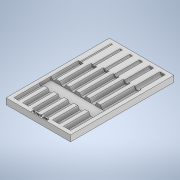
# Autodesk Inventor part: punchTray
Saved by Autodesk Inventor 2020.2 (Build 242310000, 310)
## iProperties
Created: 2019-12-07
Part Number: punchTray
Material: Generic
Document SubType Name: Modeling
Designer: robst
Density: 1 g/cm^3
Appearance: Default
Author: robst
Autodesk Inventor part; units mm, degrees
(part 1 of 2)
ref_plane "YZ Plane" through (0, 0, 0) normal (1, 0, 0) x (0, 1, 0)
ref_plane "XZ Plane" through (0, 0, 0) normal (0, 1, 0) x (-1, 0, 0)
ref_plane "XY Plane" through (0, 0, 0) normal (0, 0, 1) x (1, 0, 0)
sketch "Sketch3" plane through (0, 0, 0) normal (0, 0, 1) x (1, 0, 0)
  line L0 (-52.4636, -4.8895) -> (52.4636, -4.8895)
  line L1 (52.4636, -4.8895) -> (52.4636, 4.8895)
  line L2 (52.4636, 4.8895) -> (-52.4636, 4.8895)
  line L3 (-52.4636, 4.8895) -> (-52.4636, -4.8895)
  line L4 (-52.4636, -4.8895) -> (52.4636, 4.8895) construction
  line L5 (52.4636, -4.8895) -> (-52.4636, 4.8895) construction
  line L6 (46.1136, 4.8895) -> (43.2173, -0.127)
  line L7 (43.2173, -0.127) -> (37.4248, -0.127)
  line L8 (37.4248, -0.127) -> (34.5285, 4.8895)
  line L9 (34.5285, 4.8895) -> (37.4248, 9.906)
  line L10 (37.4248, 9.906) -> (43.2173, 9.906)
  line L11 (43.2173, 9.906) -> (46.1136, 4.8895)
  line L12 (28.1785, 4.8895) -> (25.2822, -0.127)
  line L13 (25.2822, -0.127) -> (19.4897, -0.127)
  line L14 (19.4897, -0.127) -> (16.5934, 4.8895)
  line L15 (16.5934, 4.8895) -> (19.4897, 9.906)
  line L16 (19.4897, 9.906) -> (25.2822, 9.906)
  line L17 (25.2822, 9.906) -> (28.1785, 4.8895)
  line L18 (0, 0) -> (0, 4.8895) construction
  line L19 (10.2434, 4.8895) -> (7.787, 0.635)
  line L20 (7.787, 0.635) -> (2.8744, 0.635)
  line L21 (2.8744, 0.635) -> (0.418, 4.8895)
  line L22 (0.418, 4.8895) -> (2.8744, 9.144)
  line L23 (2.8744, 9.144) -> (7.787, 9.144)
  line L24 (7.787, 9.144) -> (10.2434, 4.8895)
  line L25 (-5.932, 4.8895) -> (-8.3883, 0.635)
  line L26 (-8.3883, 0.635) -> (-13.301, 0.635)
  line L27 (-13.301, 0.635) -> (-15.7573, 4.8895)
  line L28 (-15.7573, 4.8895) -> (-13.301, 9.144)
  line L29 (-13.301, 9.144) -> (-8.3883, 9.144)
  line L30 (-8.3883, 9.144) -> (-5.932, 4.8895)
  line L31 (-22.1073, 4.8895) -> (-24.5416, 0.6731)
  line L32 (-24.5416, 0.6731) -> (-29.4103, 0.6731)
  line L33 (-29.4103, 0.6731) -> (-31.8447, 4.8895)
  line L34 (-31.8447, 4.8895) -> (-29.4103, 9.1059)
  line L35 (-29.4103, 9.1059) -> (-24.5416, 9.1059)
  line L36 (-24.5416, 9.1059) -> (-22.1073, 4.8895)
  line L37 (-38.1947, 4.8895) -> (-40.1744, 1.4605)
  line L38 (-40.1744, 1.4605) -> (-44.1339, 1.4605)
  line L39 (-44.1339, 1.4605) -> (-46.1136, 4.8895)
  line L40 (-46.1136, 4.8895) -> (-44.1339, 8.3185)
  line L41 (-44.1339, 8.3185) -> (-40.1744, 8.3185)
  line L42 (-40.1744, 8.3185) -> (-38.1947, 4.8895)
  point P0 (40.321, 4.8895)
  point P1 (22.3859, 4.8895)
  point P2 (34.5285, 4.8895)
  point P3 (16.5934, 4.8895)
  point P4 (5.3307, 4.8895)
  point P5 (-10.8446, 4.8895)
  point P6 (-26.976, 4.8895)
  point P7 (-42.1541, 4.8895)
  point P8 (0.418, 4.8895)
  point P9 (-15.7573, 4.8895)
  point P10 (-31.8447, 4.8895)
  point P11 (-46.1136, 4.8895)
  dimension "d7" = 10.033
  dimension "d8" = 10.033
  dimension "d13" = 6.35
  dimension "d14" = 6.35
  dimension "d15" = 8.509
  dimension "d16" = 6.35
  dimension "d17" = 8.509
  dimension "d18" = 6.35
  dimension "d19" = 8.4328
  dimension "d20" = 6.35
  dimension "d21" = 6.35
  dimension "d22" = 6.858
  dimension "d23" = 6.35
  dimension "d24" = 4.7625
  constraints: 84 end point, 2 horizontal, 2 midpoint, 1 parallel, 1 perpendicular, 94 other
  measures "d7" distance between parallel lines of L7 L10
  measures "d8" distance between parallel lines of L13 L16
  measures "d13" distance of L6.start L1.end
  measures "d14" distance of L8.end L12.start
  measures "d15" distance between parallel lines of L20 L23
  measures "d16" distance of L14.end L19.start
  measures "d17" distance between parallel lines of L26 L29
  measures "d18" distance of L21.end L25.start
  measures "d19" distance between parallel lines of L32 L35
  measures "d20" distance of L27.end L31.start
  measures "d21" distance of L33.end L37.start
  measures "d22" distance between parallel lines of L38 L41
  measures "d23" distance from line of L39.end L3
  measures "d24" distance between parallel lines of L0 L7
extrude "Extrusion3" add sketch "Sketch3" against normal blind 155.575 contours L3 L2 L39 L38 L37 L33 L32 L31 L27 L26 L25 L21 L20 L19 L14 L13 L12 L8 L7 L6 L1 L0
sketch "Sketch4" plane through (0, 0, 0) normal (0, 0, 1) x (1, 0, 0)
  line L0 (52.4636, -4.8895) -> (-52.4636, -4.8895) projected
  line L1 (52.4636, 4.8895) -> (52.4636, -4.8895) projected
  line L2 (-52.4636, -4.8895) -> (52.4636, -4.8895)
  line L3 (52.4636, -4.8895) -> (52.4636, 4.8895)
  line L4 (52.4636, 4.8895) -> (-52.4636, 4.8895)
  line L5 (-52.4636, 4.8895) -> (-52.4636, -4.8895)
  point P0 (0, 0)
  constraints: 8 end point, 2 parallel, 1 horizontal, 1 perpendicular
extrude "Extrusion4" add sketch "Sketch4" along normal blind 6.35
sketch "Sketch6" plane through (0, 0, -155.575) normal (0, 0, -1) x (-1, 0, 0)
  line L0 (-37.4248, -0.127) -> (-43.2173, -0.127) construction
  line L1 (-40.321, -0.127) -> (-40.321, 4.8895) construction
  line L2 (-52.4636, 4.8895) -> (52.4636, 4.8895) construction
  arc A0 (-44.5438, 4.8895) -> (-36.0983, 4.8895) centre (-40.321, 4.8895) ccw
  line L3 (-34.5285, 4.8895) -> (-37.4248, -0.127)
  line L4 (-37.4248, -0.127) -> (-43.2173, -0.127)
  line L5 (-43.2173, -0.127) -> (-46.1136, 4.8895)
  line L6 (-46.1136, 4.8895) -> (-44.5438, 4.8895)
  line L7 (-34.5285, 4.8895) -> (-36.0983, 4.8895)
  point P0 (0, 0)
  dimension "d31" = 8.4455
  constraints: 12 end point, 3 point on line, 2 coincident, 2 point on circle, 1 centre point, 1 midpoint, 1 vertical, 6 other
  measures "d31" diameter of A0
extrude "5_16_punch" add sketch "Sketch6" against normal blind 40.64
sketch "Sketch7" plane through (0, 0, -155.575) normal (0, 0, -1) x (-1, 0, 0)
  line L0 (-28.1785, 4.8895) -> (-16.5934, 4.8895) projected
  line L1 (-16.5934, 4.8895) -> (-19.4897, -0.127)
  line L2 (-19.4897, -0.127) -> (-25.2822, -0.127)
  line L3 (-25.2822, -0.127) -> (-28.1785, 4.8895)
  arc A0 (-25.8149, 4.8895) -> (-18.9569, 4.8895) centre (-22.3859, 4.8895) ccw
  line L4 (-28.1785, 4.8895) -> (-25.8149, 4.8895)
  line L5 (-10.2434, 4.8895) -> (-16.5934, 4.8895) projected
  line L6 (-16.5934, 4.8895) -> (-18.9569, 4.8895)
  point P0 (0, 0)
  point P1 (-28.1785, 4.8895)
  dimension "d34" = 6.858
  constraints: 10 end point, 2 point on circle, 2 point on line, 1 centre point, 1 coincident, 1 midpoint, 6 other
  measures "d34" diameter of A0
extrude "1_4_punch" add sketch "Sketch7" against normal blind 40.64 contours L0 A0 L1 L2 L3
sketch "Sketch8" plane through (0, 0, -155.575) normal (0, 0, -1) x (-1, 0, 0)
  line L0 (-10.2434, 4.8895) -> (-0.418, 4.8895) projected
  line L1 (-0.418, 4.8895) -> (-2.8744, 0.635)
  line L2 (-2.8744, 0.635) -> (-7.787, 0.635)
  line L3 (-7.787, 0.635) -> (-10.2434, 4.8895)
  arc A0 (-7.966, 4.8895) -> (-2.6955, 4.8895) centre (-5.3307, 4.8895) ccw
  line L4 (-10.2434, 4.8895) -> (-7.787, 0.635) projected
  line L5 (-10.2434, 4.8895) -> (-7.966, 4.8895)
  line L6 (-0.418, 4.8895) -> (-2.6955, 4.8895)
  point P0 (0, 0)
  dimension "d37" = 5.2705
  constraints: 10 end point, 2 point on circle, 2 point on line, 1 centre point, 1 coincident, 1 midpoint, 6 other
  measures "d37" diameter of A0
extrude "3_16_punch" add sketch "Sketch8" against normal blind 40.64 contours L0 A0 L1 L2 L3
sketch "Sketch9" plane through (0, 0, -155.575) normal (0, 0, -1) x (-1, 0, 0)
  line L0 (13.301, 0.635) -> (8.3883, 0.635) construction
  line L1 (10.8446, 0.635) -> (10.8446, 4.8895) construction
  line L2 (-52.4636, 4.8895) -> (52.4636, 4.8895) construction
  line L3 (15.7573, 4.8895) -> (13.301, 0.635) projected
  line L4 (15.7573, 4.8895) -> (13.301, 0.635)
  line L5 (13.301, 0.635) -> (8.3883, 0.635)
  line L6 (8.3883, 0.635) -> (5.932, 4.8895)
  arc A0 (8.6063, 4.8895) -> (13.083, 4.8895) centre (10.8446, 4.8895) ccw
  line L7 (8.3883, 0.635) -> (5.932, 4.8895) projected
  line L8 (5.932, 4.8895) -> (8.6063, 4.8895)
  line L9 (22.1073, 4.8895) -> (15.7573, 4.8895) projected
  line L10 (15.7573, 4.8895) -> (13.083, 4.8895)
  point P0 (0, 0)
  point P1 (13.301, 0.635)
  dimension "d40" = 4.4768
  constraints: 12 end point, 3 point on line, 2 coincident, 2 point on circle, 1 centre point, 1 midpoint, 1 vertical, 6 other
  measures "d40" diameter of A0
extrude "5_32_punch" add sketch "Sketch9" against normal blind 40.64
sketch "Sketch11" plane through (0, 0, -155.575) normal (0, 0, -1) x (-1, 0, 0)
  line L0 (22.1073, 4.8895) -> (31.8447, 4.8895) projected
  line L1 (29.4103, 0.6731) -> (31.8447, 4.8895) projected
  line L2 (31.8447, 4.8895) -> (29.4103, 0.6731)
  line L3 (29.4103, 0.6731) -> (24.5416, 0.6731)
  line L4 (24.5416, 0.6731) -> (22.1073, 4.8895)
  arc A0 (25.1345, 4.8895) -> (28.8175, 4.8895) centre (26.976, 4.8895) ccw
  line L5 (22.1073, 4.8895) -> (24.5416, 0.6731) projected
  line L6 (22.1073, 4.8895) -> (25.1345, 4.8895)
  line L7 (31.8447, 4.8895) -> (28.8175, 4.8895)
  point P0 (0, 0)
  point P1 (29.4103, 0.6731)
  point P2 (22.1073, 4.8895)
  dimension "d44" = 3.683
  constraints: 10 end point, 2 point on circle, 2 point on line, 1 centre point, 1 coincident, 1 midpoint, 6 other
  measures "d44" diameter of A0
extrude "1_8_punch" add sketch "Sketch11" against normal blind 44.45 contours L0 A0 L1 L3 L4
sketch "Sketch12" plane through (0, 0, -155.575) normal (0, 0, -1) x (-1, 0, 0)
  line L0 (40.1744, 1.4605) -> (44.1339, 1.4605) construction
  line L1 (42.1541, 1.4605) -> (42.1541, 4.8895) construction
  line L2 (-52.4636, 4.8895) -> (52.4636, 4.8895) construction
  line L3 (44.1339, 1.4605) -> (46.1136, 4.8895) projected
  line L4 (46.1136, 4.8895) -> (44.1339, 1.4605)
  line L5 (44.1339, 1.4605) -> (40.1744, 1.4605)
  line L6 (40.1744, 1.4605) -> (38.1947, 4.8895)
  arc A0 (41.1064, 4.8895) -> (43.2019, 4.8895) centre (42.1541, 4.8895) ccw
  line L7 (38.1947, 4.8895) -> (28.8175, 4.8895) projected
  line L8 (38.1947, 4.8895) -> (41.1064, 4.8895)
  line L9 (46.1136, 4.8895) -> (43.2019, 4.8895)
  point P0 (0, 0)
  point P1 (44.1339, 1.4605)
  dimension "d47" = 2.0955
  constraints: 12 end point, 3 point on line, 2 coincident, 2 point on circle, 1 centre point, 1 midpoint, 1 vertical, 6 other
  measures "d47" diameter of A0
extrude "1_16_punch" add sketch "Sketch12" against normal blind 50.8
sketch "Sketch5" plane through (0, 0, -155.575) normal (0, 0, -1) x (-1, 0, 0)
  line L0 (-52.4636, 4.8895) -> (-52.4636, -4.8895) projected
  line L1 (52.4636, 4.8895) -> (46.1136, 4.8895) projected
  line L2 (-52.4636, -4.8895) -> (52.4636, -4.8895)
  line L3 (52.4636, -4.8895) -> (52.4636, 4.8895)
  line L4 (52.4636, 4.8895) -> (-52.4636, 4.8895)
  line L5 (-52.4636, 4.8895) -> (-52.4636, -4.8895)
  point P0 (0, 0)
  constraints: 8 end point, 2 parallel, 1 horizontal, 1 perpendicular
extrude "Extrusion5" add sketch "Sketch5" along normal blind 6.35
sketch "Sketch13" plane through (-52.4636, 4.8895, 6.35) normal (0, 1, 0) x (1, 0, 0)
  line L0 (6.35, 6.35) -> (6.35, 111.125) projected
  line L1 (98.5772, 6.35) -> (98.5772, 121.285) projected
  line L2 (6.35, 47.625) -> (98.5772, 47.625)
  line L3 (98.5772, 47.625) -> (98.5772, 66.675)
  line L4 (98.5772, 66.675) -> (6.35, 66.675)
  line L5 (6.35, 66.675) -> (6.35, 47.625)
  line L6 (6.35, 57.15) -> (98.5772, 57.15) construction
  line L7 (14.2689, 6.35) -> (6.35, 6.35) construction
  point P0 (52.4636, 6.35)
  point P1 (6.35, 66.675)
  dimension "d50" = 19.05
  dimension "d51" = 50.8
  constraints: 10 end point, 2 midpoint, 2 parallel, 2 point on line, 1 horizontal, 1 perpendicular
  measures "d50" distance between parallel lines of L4 L2
  measures "d51" distance between parallel lines of L6 L7
extrude "Extrusion12" cut sketch "Sketch13" against normal blind 5.08
sketch "Sketch14" plane through (-52.4636, 4.8895, 6.35) normal (0, 1, 0) x (1, 0, 0)
  line L0 (0, 168.275) -> (0, 0) construction
  line L1 (0, 3.175) -> (104.9272, 3.175) construction
  line L2 (0, 0) -> (104.9272, 0) construction
  spline S0 degree 2 poles (42.5851, 3.879) (42.5851, 3.6134) (42.4153, 3.1318) (42.2578, 2.9712) knots 0 0 0 1 2 2 2
  spline S1 degree 2 poles (42.2578, 2.9712) (42.1621, 2.8693) (41.9274, 2.7026) (41.7885, 2.6439) knots 0 0 0 1 2 2 2
  spline S2 degree 2 poles (41.7885, 2.6439) (41.6465, 2.5853) (41.3161, 2.5174) (41.1123, 2.5174) knots 0 0 0 1 2 2 2
  line L3 (41.1123, 2.5174) -> (40.6122, 2.5174)
  line L4 (40.6122, 2.5174) -> (40.6122, 1.27)
  line L5 (40.6122, 1.27) -> (39.655, 1.27)
  line L6 (39.655, 1.27) -> (39.655, 5.08)
  line L7 (39.655, 5.08) -> (41.1339, 5.08)
  spline S3 degree 2 poles (41.1339, 5.08) (41.4612, 5.08) (41.9398, 4.9596) (42.1343, 4.8299) knots 0 0 0 1 2 2 2
  spline S4 degree 2 poles (42.1343, 4.8299) (42.3504, 4.6848) (42.5851, 4.2093) (42.5851, 3.879) knots 0 0 0 1 2 2 2
  spline S5 degree 2 poles (41.6033, 3.8543) (41.6033, 4.0179) (41.4489, 4.2495) (41.3439, 4.2927) knots 0 0 0 1 2 2 2
  spline S6 degree 2 poles (41.3439, 4.2927) (41.208, 4.3513) (40.961, 4.3699) (40.748, 4.3699) knots 0 0 0 1 2 2 2
  line L8 (40.748, 4.3699) -> (40.6122, 4.3699)
  line L9 (40.6122, 4.3699) -> (40.6122, 3.2275)
  line L10 (40.6122, 3.2275) -> (40.6801, 3.2275)
  spline S7 degree 2 poles (40.6801, 3.2275) (40.8128, 3.2275) (41.0537, 3.2337) (41.1432, 3.2491) knots 0 0 0 1 2 2 2
  spline S8 degree 2 poles (41.1432, 3.2491) (41.2204, 3.2615) (41.3902, 3.3356) (41.4365, 3.3819) knots 0 0 0 1 2 2 2
  spline S9 degree 2 poles (41.4365, 3.3819) (41.5353, 3.4745) (41.6033, 3.6814) (41.6033, 3.8543) knots 0 0 0 1 2 2 2
  line L11 (45.7127, 1.27) -> (44.8174, 1.27)
  line L12 (44.8174, 1.27) -> (44.8174, 1.588)
  spline S10 degree 2 poles (44.8174, 1.588) (44.5858, 1.3935) (44.1968, 1.1897) (43.9282, 1.1897) knots 0 0 0 1 2 2 2
  spline S11 degree 2 poles (43.9282, 1.1897) (43.5021, 1.1897) (43.0235, 1.73) (43.0235, 2.2734) knots 0 0 0 1 2 2 2
  line L13 (43.0235, 2.2734) -> (43.0235, 4.1445)
  line L14 (43.0235, 4.1445) -> (43.9251, 4.1445)
  line L15 (43.9251, 4.1445) -> (43.9251, 2.718)
  spline S12 degree 2 poles (43.9251, 2.718) (43.9251, 2.4957) (43.9467, 2.2117) (43.9899, 2.116) knots 0 0 0 1 2 2 2
  spline S13 degree 2 poles (43.9899, 2.116) (44.0331, 2.0264) (44.2029, 1.9338) (44.3573, 1.9338) knots 0 0 0 1 2 2 2
  spline S14 degree 2 poles (44.3573, 1.9338) (44.4499, 1.9338) (44.7093, 2.0264) (44.8174, 2.1067) knots 0 0 0 1 2 2 2
  line L16 (44.8174, 2.1067) -> (44.8174, 4.1445)
  line L17 (44.8174, 4.1445) -> (45.7127, 4.1445)
  line L18 (45.7127, 4.1445) -> (45.7127, 1.27)
  line L19 (49.0874, 1.27) -> (48.1858, 1.27)
  line L20 (48.1858, 1.27) -> (48.1858, 2.6933)
  spline S15 degree 2 poles (48.1858, 2.6933) (48.1858, 2.8693) (48.1581, 3.2151) (48.121, 3.2954) knots 0 0 0 1 2 2 2
  spline S16 degree 2 poles (48.121, 3.2954) (48.0747, 3.3942) (47.9018, 3.4776) (47.7536, 3.4776) knots 0 0 0 1 2 2 2
  spline S17 degree 2 poles (47.7536, 3.4776) (47.6455, 3.4776) (47.4201, 3.3942) (47.2936, 3.3047) knots 0 0 0 1 2 2 2
  line L21 (47.2936, 3.3047) -> (47.2936, 1.27)
  line L22 (47.2936, 1.27) -> (46.3982, 1.27)
  line L23 (46.3982, 1.27) -> (46.3982, 4.1445)
  line L24 (46.3982, 4.1445) -> (47.2936, 4.1445)
  line L25 (47.2936, 4.1445) -> (47.2936, 3.8265)
  spline S18 degree 2 poles (47.2936, 3.8265) (47.5128, 4.0117) (47.9296, 4.2217) (48.1828, 4.2217) knots 0 0 0 1 2 2 2
  spline S19 degree 2 poles (48.1828, 4.2217) (48.6212, 4.2217) (49.0874, 3.6659) (49.0874, 3.141) knots 0 0 0 1 2 2 2
  line L26 (49.0874, 3.141) -> (49.0874, 1.27)
  spline S20 degree 2 poles (51.1591, 1.1928) (50.8041, 1.1928) (50.2143, 1.3719) (49.9951, 1.5571) knots 0 0 0 1 2 2 2
  spline S21 degree 2 poles (49.9951, 1.5571) (49.7821, 1.7455) (49.5413, 2.3105) (49.5413, 2.6933) knots 0 0 0 1 2 2 2
  spline S22 degree 2 poles (49.5413, 2.6933) (49.5413, 3.1071) (49.8006, 3.6844) (50.026, 3.8697) knots 0 0 0 1 2 2 2
  spline S23 degree 2 poles (50.026, 3.8697) (50.239, 4.0488) (50.8195, 4.2217) (51.1344, 4.2217) knots 0 0 0 1 2 2 2
  spline S24 degree 2 poles (51.1344, 4.2217) (51.3722, 4.2217) (51.8476, 4.1105) (52.0885, 3.9901) knots 0 0 0 1 2 2 2
  line L27 (52.0885, 3.9901) -> (52.0885, 3.2244)
  line L28 (52.0885, 3.2244) -> (51.9742, 3.2244)
  spline S25 degree 2 poles (51.9742, 3.2244) (51.9187, 3.2769) (51.7643, 3.4004) (51.6717, 3.4498) knots 0 0 0 1 2 2 2
  spline S26 degree 2 poles (51.6717, 3.4498) (51.5729, 3.5054) (51.3289, 3.5795) (51.1777, 3.5795) knots 0 0 0 1 2 2 2
  spline S27 degree 2 poles (51.1777, 3.5795) (50.8349, 3.5795) (50.4583, 3.1009) (50.4583, 2.6933) knots 0 0 0 1 2 2 2
  spline S28 degree 2 poles (50.4583, 2.6933) (50.4583, 2.2611) (50.8596, 1.835) (51.1931, 1.835) knots 0 0 0 1 2 2 2
  spline S29 degree 2 poles (51.1931, 1.835) (51.3629, 1.835) (51.6161, 1.9122) (51.7087, 1.9678) knots 0 0 0 1 2 2 2
  spline S30 degree 2 poles (51.7087, 1.9678) (51.7982, 2.0203) (51.9279, 2.1376) (51.9742, 2.1839) knots 0 0 0 1 2 2 2
  line L29 (51.9742, 2.1839) -> (52.0885, 2.1839)
  line L30 (52.0885, 2.1839) -> (52.0885, 1.4151)
  spline S31 degree 2 poles (52.0885, 1.4151) (52.0113, 1.3812) (51.8106, 1.2947) (51.7056, 1.2669) knots 0 0 0 1 2 2 2
  spline S32 degree 2 poles (51.7056, 1.2669) (51.5759, 1.2299) (51.3475, 1.1928) (51.1591, 1.1928) knots 0 0 0 1 2 2 2
  line L31 (55.2038, 1.27) -> (54.3022, 1.27)
  line L32 (54.3022, 1.27) -> (54.3022, 2.6933)
  spline S33 degree 2 poles (54.3022, 2.6933) (54.3022, 2.8693) (54.2744, 3.2151) (54.2374, 3.2954) knots 0 0 0 1 2 2 2
  spline S34 degree 2 poles (54.2374, 3.2954) (54.1911, 3.3942) (54.0182, 3.4776) (53.87, 3.4776) knots 0 0 0 1 2 2 2
  spline S35 degree 2 poles (53.87, 3.4776) (53.7619, 3.4776) (53.5365, 3.3942) (53.4099, 3.3047) knots 0 0 0 1 2 2 2
  line L33 (53.4099, 3.3047) -> (53.4099, 1.27)
  line L34 (53.4099, 1.27) -> (52.5145, 1.27)
  line L35 (52.5145, 1.27) -> (52.5145, 5.2498)
  line L36 (52.5145, 5.2498) -> (53.4099, 5.2498)
  line L37 (53.4099, 5.2498) -> (53.4099, 3.8265)
  spline S36 degree 2 poles (53.4099, 3.8265) (53.6291, 4.0117) (54.046, 4.2217) (54.2991, 4.2217) knots 0 0 0 1 2 2 2
  spline S37 degree 2 poles (54.2991, 4.2217) (54.7376, 4.2217) (55.2038, 3.6659) (55.2038, 3.141) knots 0 0 0 1 2 2 2
  line L38 (55.2038, 3.141) -> (55.2038, 1.27)
  spline S38 degree 2 poles (58.6309, 1.2021) (58.1925, 1.2021) (57.5318, 1.3719) (57.2477, 1.4954) knots 0 0 0 1 2 2 2
  line L39 (57.2477, 1.4954) -> (57.2477, 2.4031)
  line L40 (57.2477, 2.4031) -> (57.3342, 2.4031)
  spline S39 degree 2 poles (57.3342, 2.4031) (57.6213, 2.1592) (58.3098, 1.8968) (58.634, 1.8968) knots 0 0 0 1 2 2 2
  spline S40 degree 2 poles (58.634, 1.8968) (58.7174, 1.8968) (58.986, 1.9338) (59.0663, 1.9709) knots 0 0 0 1 2 2 2
  spline S41 degree 2 poles (59.0663, 1.9709) (59.1651, 2.0141) (59.304, 2.1716) (59.304, 2.2981) knots 0 0 0 1 2 2 2
  spline S42 degree 2 poles (59.304, 2.2981) (59.304, 2.4433) (59.0786, 2.6223) (58.9242, 2.6625) knots 0 0 0 1 2 2 2
  spline S43 degree 2 poles (58.9242, 2.6625) (58.7297, 2.715) (58.2882, 2.8045) (58.0937, 2.8724) knots 0 0 0 1 2 2 2
  spline S44 degree 2 poles (58.0937, 2.8724) (57.6522, 3.0268) (57.2693, 3.5548) (57.2693, 3.95) knots 0 0 0 1 2 2 2
  spline S45 degree 2 poles (57.2693, 3.95) (57.2693, 4.4841) (58.174, 5.1479) (58.8532, 5.1479) knots 0 0 0 1 2 2 2
  spline S46 degree 2 poles (58.8532, 5.1479) (59.1929, 5.1479) (59.8659, 5.009) (60.1315, 4.8917) knots 0 0 0 1 2 2 2
  line L41 (60.1315, 4.8917) -> (60.1315, 4.021)
  line L42 (60.1315, 4.021) -> (60.0481, 4.021)
  spline S47 degree 2 poles (60.0481, 4.021) (59.8351, 4.2031) (59.2237, 4.4532) (58.9026, 4.4532) knots 0 0 0 1 2 2 2
  spline S48 degree 2 poles (58.9026, 4.4532) (58.776, 4.4532) (58.5784, 4.4162) (58.4673, 4.3668) knots 0 0 0 1 2 2 2
  spline S49 degree 2 poles (58.4673, 4.3668) (58.3778, 4.3266) (58.2481, 4.1661) (58.2481, 4.0673) knots 0 0 0 1 2 2 2
  spline S50 degree 2 poles (58.2481, 4.0673) (58.2481, 3.9191) (58.4549, 3.7493) (58.7513, 3.6814) knots 0 0 0 1 2 2 2
  spline S51 degree 2 poles (58.7513, 3.6814) (58.9428, 3.6381) (59.2978, 3.5548) (59.5016, 3.4838) knots 0 0 0 1 2 2 2
  spline S52 degree 2 poles (59.5016, 3.4838) (59.8968, 3.3386) (60.2828, 2.857) (60.2828, 2.4618) knots 0 0 0 1 2 2 2
  spline S53 degree 2 poles (60.2828, 2.4618) (60.2828, 1.8937) (59.3905, 1.2021) (58.6309, 1.2021) knots 0 0 0 1 2 2 2
  spline S54 degree 2 poles (62.1939, 1.1928) (61.3788, 1.1928) (60.5112, 1.9709) (60.5112, 2.6903) knots 0 0 0 1 2 2 2
  spline S55 degree 2 poles (60.5112, 2.6903) (60.5112, 3.3942) (61.3202, 4.234) (62.0488, 4.234) knots 0 0 0 1 2 2 2
  spline S56 degree 2 poles (62.0488, 4.234) (62.7065, 4.234) (63.3734, 3.5208) (63.3734, 2.8601) knots 0 0 0 1 2 2 2
  line L43 (63.3734, 2.8601) -> (63.3734, 2.5359)
  line L44 (63.3734, 2.5359) -> (61.4066, 2.5359)
  spline S57 degree 2 poles (61.4066, 2.5359) (61.419, 2.3352) (61.5641, 2.0697) (61.6814, 1.9894) knots 0 0 0 1 2 2 2
  spline S58 degree 2 poles (61.6814, 1.9894) (61.7956, 1.9091) (62.1044, 1.8412) (62.2866, 1.8412) knots 0 0 0 1 2 2 2
  spline S59 degree 2 poles (62.2866, 1.8412) (62.4409, 1.8412) (62.7435, 1.9091) (62.8701, 1.9678) knots 0 0 0 1 2 2 2
  spline S60 degree 2 poles (62.8701, 1.9678) (62.9812, 2.0141) (63.1665, 2.1283) (63.2252, 2.1716) knots 0 0 0 1 2 2 2
  line L45 (63.2252, 2.1716) -> (63.3209, 2.1716)
  line L46 (63.3209, 2.1716) -> (63.3209, 1.4306)
  spline S61 degree 2 poles (63.3209, 1.4306) (63.2097, 1.3873) (63.0306, 1.3132) (62.8701, 1.2762) knots 0 0 0 1 2 2 2
  spline S62 degree 2 poles (62.8701, 1.2762) (62.725, 1.236) (62.4162, 1.1928) (62.1939, 1.1928) knots 0 0 0 1 2 2 2
  spline S63 degree 2 poles (62.4903, 3.0762) (62.4842, 3.3603) (62.2341, 3.6597) (61.9778, 3.6597) knots 0 0 0 1 2 2 2
  spline S64 degree 2 poles (61.9778, 3.6597) (61.7154, 3.6597) (61.419, 3.3448) (61.4035, 3.0762) knots 0 0 0 1 2 2 2
  line L47 (61.4035, 3.0762) -> (62.4903, 3.0762)
  spline S65 degree 2 poles (64.9326, 1.2144) (64.3861, 1.2144) (63.8859, 1.6652) (63.8859, 2.1777) knots 0 0 0 1 2 2 2
  line L48 (63.8859, 2.1777) -> (63.8859, 3.5208)
  line L49 (63.8859, 3.5208) -> (63.5432, 3.5208)
  line L50 (63.5432, 3.5208) -> (63.5432, 4.1445)
  line L51 (63.5432, 4.1445) -> (63.8859, 4.1445)
  line L52 (63.8859, 4.1445) -> (63.8859, 4.9658)
  line L53 (63.8859, 4.9658) -> (64.7813, 4.9658)
  line L54 (64.7813, 4.9658) -> (64.7813, 4.1445)
  line L55 (64.7813, 4.1445) -> (65.6458, 4.1445)
  line L56 (65.6458, 4.1445) -> (65.6458, 3.5208)
  line L57 (65.6458, 3.5208) -> (64.7813, 3.5208)
  line L58 (64.7813, 3.5208) -> (64.7813, 2.4988)
  spline S66 degree 2 poles (64.7813, 2.4988) (64.7813, 2.3475) (64.7874, 2.1222) (64.8245, 2.0326) knots 0 0 0 1 2 2 2
  spline S67 degree 2 poles (64.8245, 2.0326) (64.8615, 1.9431) (65.0437, 1.8381) (65.2166, 1.8381) knots 0 0 0 1 2 2 2
  spline S68 degree 2 poles (65.2166, 1.8381) (65.2907, 1.8381) (65.5223, 1.8999) (65.5686, 1.9246) knots 0 0 0 1 2 2 2
  line L59 (65.5686, 1.9246) -> (65.6458, 1.9246)
  line L60 (65.6458, 1.9246) -> (65.6458, 1.2947)
  spline S69 degree 2 poles (65.6458, 1.2947) (65.5007, 1.2576) (65.1734, 1.2144) (64.9326, 1.2144) knots 0 0 0 1 2 2 2
  point P0 (52.4636, 6.35)
  dimension "d54" = 3.175
  constraints: 2 end point, 1 horizontal, 1 parallel, 1 point on line
  measures "d54" distance between parallel lines of L1 L2
extrude "Extrusion13" cut sketch "Sketch14" against normal blind 3.175
sketch "Sketch15" plane through (-52.4636, -4.8895, 6.35) normal (0, -1, 0) x (1, 0, 0)
  line L0 (104.9272, -168.275) -> (104.9272, 0) construction
  line L1 (104.9272, -84.1375) -> (0, -84.1375) construction
  line L2 (0, -168.275) -> (0, 0) construction
  spline S0 degree 2 poles (77.1638, -95.5613) (77.1638, -94.493) (78.0962, -92.8134) (78.8063, -92.3627) knots 0 0 0 1 2 2 2
  spline S1 degree 2 poles (78.8063, -92.3627) (79.3991, -91.9798) (80.7947, -91.7575) (81.5789, -91.7575) knots 0 0 0 1 2 2 2
  line L3 (81.5789, -91.7575) -> (83.9625, -91.7575)
  line L4 (83.9625, -91.7575) -> (83.9625, -99.3775)
  line L5 (83.9625, -99.3775) -> (81.6036, -99.3775)
  spline S2 degree 2 poles (81.6036, -99.3775) (80.8009, -99.3775) (79.3991, -99.1737) (78.7816, -98.7785) knots 0 0 0 1 2 2 2
  spline S3 degree 2 poles (78.7816, -98.7785) (78.0344, -98.2969) (77.1638, -96.6667) (77.1638, -95.5613) knots 0 0 0 1 2 2 2
  spline S4 degree 2 poles (79.1274, -95.5737) (79.1274, -96.327) (79.6461, -97.4015) (80.1772, -97.7041) knots 0 0 0 1 2 2 2
  spline S5 degree 2 poles (80.1772, -97.7041) (80.5662, -97.914) (81.4184, -97.9572) (82.0112, -97.9572) knots 0 0 0 1 2 2 2
  line L6 (82.0112, -97.9572) -> (82.0482, -97.9572)
  line L7 (82.0482, -97.9572) -> (82.0482, -93.1839)
  line L8 (82.0482, -93.1839) -> (82.0112, -93.1839)
  spline S6 degree 2 poles (82.0112, -93.1839) (81.369, -93.1839) (80.4859, -93.2272) (80.0846, -93.4803) knots 0 0 0 1 2 2 2
  spline S7 degree 2 poles (80.0846, -93.4803) (79.6153, -93.7767) (79.1274, -94.8203) (79.1274, -95.5737) knots 0 0 0 1 2 2 2
  spline S8 degree 2 poles (73.187, -91.6031) (74.8173, -91.6031) (76.5524, -93.1592) (76.5524, -94.598) knots 0 0 0 1 2 2 2
  spline S9 degree 2 poles (76.5524, -94.598) (76.5524, -96.0059) (74.9346, -97.6855) (73.4773, -97.6855) knots 0 0 0 1 2 2 2
  spline S10 degree 2 poles (73.4773, -97.6855) (72.162, -97.6855) (70.8282, -96.2591) (70.8282, -94.9376) knots 0 0 0 1 2 2 2
  line L9 (70.8282, -94.9376) -> (70.8282, -94.2893)
  line L10 (70.8282, -94.2893) -> (74.7617, -94.2893)
  spline S11 degree 2 poles (74.7617, -94.2893) (74.737, -93.8879) (74.4467, -93.3568) (74.2121, -93.1963) knots 0 0 0 1 2 2 2
  spline S12 degree 2 poles (74.2121, -93.1963) (73.9836, -93.0357) (73.3661, -92.8999) (73.0018, -92.8999) knots 0 0 0 1 2 2 2
  spline S13 degree 2 poles (73.0018, -92.8999) (72.693, -92.8999) (72.0879, -93.0357) (71.8347, -93.1531) knots 0 0 0 1 2 2 2
  spline S14 degree 2 poles (71.8347, -93.1531) (71.6124, -93.2457) (71.2419, -93.4742) (71.1246, -93.5606) knots 0 0 0 1 2 2 2
  line L11 (71.1246, -93.5606) -> (70.9332, -93.5606)
  line L12 (70.9332, -93.5606) -> (70.9332, -92.0786)
  spline S15 degree 2 poles (70.9332, -92.0786) (71.1555, -91.9922) (71.5136, -91.844) (71.8347, -91.7699) knots 0 0 0 1 2 2 2
  spline S16 degree 2 poles (71.8347, -91.7699) (72.1249, -91.6896) (72.7424, -91.6031) (73.187, -91.6031) knots 0 0 0 1 2 2 2
  spline S17 degree 2 poles (72.5942, -95.3699) (72.6066, -95.938) (73.1068, -96.537) (73.6193, -96.537) knots 0 0 0 1 2 2 2
  spline S18 degree 2 poles (73.6193, -96.537) (74.1442, -96.537) (74.737, -95.9071) (74.7679, -95.3699) knots 0 0 0 1 2 2 2
  line L13 (74.7679, -95.3699) -> (72.5942, -95.3699)
  spline S19 degree 2 poles (68.1606, -91.6031) (68.7904, -91.6031) (69.9204, -91.881) (70.2909, -92.0663) knots 0 0 0 1 2 2 2
  line L14 (70.2909, -92.0663) -> (70.2909, -93.5791)
  line L15 (70.2909, -93.5791) -> (70.1427, -93.5791)
  spline S20 degree 2 poles (70.1427, -93.5791) (70.0131, -93.4803) (69.6858, -93.2457) (69.3956, -93.116) knots 0 0 0 1 2 2 2
  spline S21 degree 2 poles (69.3956, -93.116) (69.1424, -92.9987) (68.5187, -92.832) (68.1482, -92.832) knots 0 0 0 1 2 2 2
  spline S22 degree 2 poles (68.1482, -92.832) (67.7715, -92.832) (67.1911, -93.0666) (67.1911, -93.3198) knots 0 0 0 1 2 2 2
  spline S23 degree 2 poles (67.1911, -93.3198) (67.1911, -93.5174) (67.4566, -93.7273) (67.8395, -93.8138) knots 0 0 0 1 2 2 2
  spline S24 degree 2 poles (67.8395, -93.8138) (68.0432, -93.8694) (68.6669, -93.9867) (68.9077, -94.0608) knots 0 0 0 1 2 2 2
  spline S25 degree 2 poles (68.9077, -94.0608) (69.587, -94.2707) (70.2662, -95.092) (70.2662, -95.7651) knots 0 0 0 1 2 2 2
  spline S26 degree 2 poles (70.2662, -95.7651) (70.2662, -96.148) (69.9143, -96.8272) (69.5685, -97.0927) knots 0 0 0 1 2 2 2
  spline S27 degree 2 poles (69.5685, -97.0927) (69.2288, -97.3521) (68.2223, -97.6608) (67.5863, -97.6608) knots 0 0 0 1 2 2 2
  spline S28 degree 2 poles (67.5863, -97.6608) (66.9811, -97.6608) (65.9684, -97.42) (65.6226, -97.2533) knots 0 0 0 1 2 2 2
  line L16 (65.6226, -97.2533) -> (65.6226, -95.796)
  line L17 (65.6226, -95.796) -> (65.7646, -95.796)
  spline S29 degree 2 poles (65.7646, -95.796) (65.8573, -95.8701) (66.2586, -96.1109) (66.4439, -96.1974) knots 0 0 0 1 2 2 2
  spline S30 degree 2 poles (66.4439, -96.1974) (66.6724, -96.2962) (67.2281, -96.432) (67.5184, -96.432) knots 0 0 0 1 2 2 2
  spline S31 degree 2 poles (67.5184, -96.432) (67.9074, -96.432) (68.4446, -96.1665) (68.4446, -95.9504) knots 0 0 0 1 2 2 2
  spline S32 degree 2 poles (68.4446, -95.9504) (68.4446, -95.7528) (68.1791, -95.5304) (67.7345, -95.4193) knots 0 0 0 1 2 2 2
  spline S33 degree 2 poles (67.7345, -95.4193) (67.506, -95.3637) (66.907, -95.2587) (66.6291, -95.1661) knots 0 0 0 1 2 2 2
  spline S34 degree 2 poles (66.6291, -95.1661) (66.0116, -94.9685) (65.3694, -94.1966) (65.3694, -93.5544) knots 0 0 0 1 2 2 2
  spline S35 degree 2 poles (65.3694, -93.5544) (65.3694, -93.1531) (65.7461, -92.4182) (66.0981, -92.1712) knots 0 0 0 1 2 2 2
  spline S36 degree 2 poles (66.0981, -92.1712) (66.4624, -91.8995) (67.4628, -91.6031) (68.1606, -91.6031) knots 0 0 0 1 2 2 2
  line L18 (62.7265, -91.7575) -> (64.5173, -91.7575)
  line L19 (64.5173, -91.7575) -> (64.5173, -97.5065)
  line L20 (64.5173, -97.5065) -> (62.7265, -97.5065)
  line L21 (62.7265, -97.5065) -> (62.7265, -91.7575)
  line L22 (62.6709, -98.3277) -> (64.5667, -98.3277)
  line L23 (64.5667, -98.3277) -> (64.5667, -99.7233)
  line L24 (64.5667, -99.7233) -> (62.6709, -99.7233)
  line L25 (62.6709, -99.7233) -> (62.6709, -98.3277)
  spline S37 degree 2 poles (56.1316, -92.4182) (56.1316, -91.6216) (56.5947, -90.504) (56.9899, -90.1952) knots 0 0 0 1 2 2 2
  spline S38 degree 2 poles (56.9899, -90.1952) (57.3913, -89.8803) (58.5028, -89.5962) (59.182, -89.5962) knots 0 0 0 1 2 2 2
  spline S39 degree 2 poles (59.182, -89.5962) (59.7563, -89.5962) (60.7876, -89.7444) (61.1642, -89.8432) knots 0 0 0 1 2 2 2
  line L26 (61.1642, -89.8432) -> (61.1642, -91.282)
  line L27 (61.1642, -91.282) -> (60.9543, -91.282)
  spline S40 degree 2 poles (60.9543, -91.282) (60.8246, -91.2326) (60.4603, -91.1091) (60.275, -91.0597) knots 0 0 0 1 2 2 2
  spline S41 degree 2 poles (60.275, -91.0597) (60.0527, -91.0041) (59.6328, -90.93) (59.4167, -90.93) knots 0 0 0 1 2 2 2
  spline S42 degree 2 poles (59.4167, -90.93) (58.9597, -90.93) (58.3546, -91.1153) (58.2002, -91.2882) knots 0 0 0 1 2 2 2
  spline S43 degree 2 poles (58.2002, -91.2882) (58.0458, -91.4673) (57.9223, -91.9489) (57.9223, -92.3194) knots 0 0 0 1 2 2 2
  line L28 (57.9223, -92.3194) -> (57.9223, -92.4244)
  spline S44 degree 2 poles (57.9223, -92.4244) (58.2249, -92.1589) (59.0153, -91.8378) (59.4352, -91.8378) knots 0 0 0 1 2 2 2
  spline S45 degree 2 poles (59.4352, -91.8378) (60.5529, -91.8378) (61.7632, -93.2889) (61.7632, -94.7771) knots 0 0 0 1 2 2 2
  spline S46 degree 2 poles (61.7632, -94.7771) (61.7632, -95.4502) (61.3927, -96.5246) (61.0593, -96.9013) knots 0 0 0 1 2 2 2
  spline S47 degree 2 poles (61.0593, -96.9013) (60.7382, -97.2656) (59.8428, -97.6608) (59.355, -97.6608) knots 0 0 0 1 2 2 2
  spline S48 degree 2 poles (59.355, -97.6608) (58.9165, -97.6608) (58.2187, -97.4385) (57.9347, -97.2533) knots 0 0 0 1 2 2 2
  line L29 (57.9347, -97.2533) -> (57.8668, -97.5065)
  line L30 (57.8668, -97.5065) -> (56.1316, -97.5065)
  line L31 (56.1316, -97.5065) -> (56.1316, -92.4182)
  line L32 (57.9223, -93.5668) -> (57.9223, -96.1727)
  spline S49 degree 2 poles (57.9223, -96.1727) (58.052, -96.2344) (58.441, -96.3147) (58.6386, -96.3147) knots 0 0 0 1 2 2 2
  spline S50 degree 2 poles (58.6386, -96.3147) (59.2809, -96.3147) (59.9292, -95.481) (59.9292, -94.7339) knots 0 0 0 1 2 2 2
  spline S51 degree 2 poles (59.9292, -94.7339) (59.9292, -94.3634) (59.8304, -93.8447) (59.7008, -93.6471) knots 0 0 0 1 2 2 2
  spline S52 degree 2 poles (59.7008, -93.6471) (59.5711, -93.4495) (59.1573, -93.2519) (58.8362, -93.2519) knots 0 0 0 1 2 2 2
  spline S53 degree 2 poles (58.8362, -93.2519) (58.5954, -93.2519) (58.1323, -93.4186) (57.9223, -93.5668) knots 0 0 0 1 2 2 2
  line L33 (49.3823, -91.7575) -> (51.1854, -91.7575)
  line L34 (51.1854, -91.7575) -> (51.1854, -94.6042)
  spline S54 degree 2 poles (51.1854, -94.6042) (51.1854, -94.9562) (51.2409, -95.6478) (51.315, -95.8083) knots 0 0 0 1 2 2 2
  spline S55 degree 2 poles (51.315, -95.8083) (51.4077, -96.0059) (51.7535, -96.1727) (52.0499, -96.1727) knots 0 0 0 1 2 2 2
  spline S56 degree 2 poles (52.0499, -96.1727) (52.266, -96.1727) (52.7168, -96.0059) (52.97, -95.8269) knots 0 0 0 1 2 2 2
  line L35 (52.97, -95.8269) -> (52.97, -91.7575)
  line L36 (52.97, -91.7575) -> (54.7607, -91.7575)
  line L37 (54.7607, -91.7575) -> (54.7607, -97.5065)
  line L38 (54.7607, -97.5065) -> (52.97, -97.5065)
  line L39 (52.97, -97.5065) -> (52.97, -96.8704)
  spline S57 degree 2 poles (52.97, -96.8704) (52.5315, -97.2409) (51.6979, -97.6608) (51.1915, -97.6608) knots 0 0 0 1 2 2 2
  spline S58 degree 2 poles (51.1915, -97.6608) (50.3147, -97.6608) (49.3823, -96.5493) (49.3823, -95.4996) knots 0 0 0 1 2 2 2
  line L40 (49.3823, -95.4996) -> (49.3823, -91.7575)
  spline S59 degree 2 poles (45.1091, -91.6031) (46.7393, -91.6031) (48.4745, -93.1592) (48.4745, -94.598) knots 0 0 0 1 2 2 2
  spline S60 degree 2 poles (48.4745, -94.598) (48.4745, -96.0059) (46.8567, -97.6855) (45.3994, -97.6855) knots 0 0 0 1 2 2 2
  spline S61 degree 2 poles (45.3994, -97.6855) (44.0841, -97.6855) (42.7503, -96.2591) (42.7503, -94.9376) knots 0 0 0 1 2 2 2
  line L41 (42.7503, -94.9376) -> (42.7503, -94.2893)
  line L42 (42.7503, -94.2893) -> (46.6838, -94.2893)
  spline S62 degree 2 poles (46.6838, -94.2893) (46.6591, -93.8879) (46.3688, -93.3568) (46.1342, -93.1963) knots 0 0 0 1 2 2 2
  spline S63 degree 2 poles (46.1342, -93.1963) (45.9057, -93.0357) (45.2882, -92.8999) (44.9239, -92.8999) knots 0 0 0 1 2 2 2
  spline S64 degree 2 poles (44.9239, -92.8999) (44.6151, -92.8999) (44.01, -93.0357) (43.7568, -93.1531) knots 0 0 0 1 2 2 2
  spline S65 degree 2 poles (43.7568, -93.1531) (43.5345, -93.2457) (43.164, -93.4742) (43.0467, -93.5606) knots 0 0 0 1 2 2 2
  line L43 (43.0467, -93.5606) -> (42.8552, -93.5606)
  line L44 (42.8552, -93.5606) -> (42.8552, -92.0786)
  spline S66 degree 2 poles (42.8552, -92.0786) (43.0775, -91.9922) (43.4357, -91.844) (43.7568, -91.7699) knots 0 0 0 1 2 2 2
  spline S67 degree 2 poles (43.7568, -91.7699) (44.047, -91.6896) (44.6645, -91.6031) (45.1091, -91.6031) knots 0 0 0 1 2 2 2
  spline S68 degree 2 poles (44.5163, -95.3699) (44.5287, -95.938) (45.0289, -96.537) (45.5414, -96.537) knots 0 0 0 1 2 2 2
  spline S69 degree 2 poles (45.5414, -96.537) (46.0663, -96.537) (46.6591, -95.9071) (46.6899, -95.3699) knots 0 0 0 1 2 2 2
  line L45 (46.6899, -95.3699) -> (44.5163, -95.3699)
  line L46 (36.6061, -91.7575) -> (38.3969, -91.7575)
  line L47 (38.3969, -91.7575) -> (38.3969, -92.3565)
  spline S70 degree 2 poles (38.3969, -92.3565) (38.5698, -92.2145) (39.0144, -91.8872) (39.1873, -91.8007) knots 0 0 0 1 2 2 2
  spline S71 degree 2 poles (39.1873, -91.8007) (39.3972, -91.7019) (39.8171, -91.5969) (40.1073, -91.5969) knots 0 0 0 1 2 2 2
  spline S72 degree 2 poles (40.1073, -91.5969) (41.0892, -91.5969) (42.2377, -93.2272) (42.2377, -94.5857) knots 0 0 0 1 2 2 2
  spline S73 degree 2 poles (42.2377, -94.5857) (42.2377, -95.339) (41.8487, -96.4444) (41.5091, -96.8519) knots 0 0 0 1 2 2 2
  spline S74 degree 2 poles (41.5091, -96.8519) (41.1942, -97.2286) (40.305, -97.6608) (39.8109, -97.6608) knots 0 0 0 1 2 2 2
  spline S75 degree 2 poles (39.8109, -97.6608) (39.3602, -97.6608) (38.7797, -97.4694) (38.3969, -97.2718) knots 0 0 0 1 2 2 2
  line L48 (38.3969, -97.2718) -> (38.3969, -99.7171)
  line L49 (38.3969, -99.7171) -> (36.6061, -99.7171)
  line L50 (36.6061, -99.7171) -> (36.6061, -91.7575)
  line L51 (38.3969, -93.3383) -> (38.3969, -96.1603)
  spline S76 degree 2 poles (38.3969, -96.1603) (38.5265, -96.2282) (38.9588, -96.3147) (39.1132, -96.3147) knots 0 0 0 1 2 2 2
  spline S77 degree 2 poles (39.1132, -96.3147) (39.7554, -96.3147) (40.4038, -95.4131) (40.4038, -94.6042) knots 0 0 0 1 2 2 2
  spline S78 degree 2 poles (40.4038, -94.6042) (40.4038, -93.752) (39.885, -92.9925) (39.3108, -92.9925) knots 0 0 0 1 2 2 2
  spline S79 degree 2 poles (39.3108, -92.9925) (39.0761, -92.9925) (38.5945, -93.1778) (38.3969, -93.3383) knots 0 0 0 1 2 2 2
  spline S80 degree 2 poles (26.5346, -94.7092) (26.5346, -93.3383) (27.924, -91.6463) (28.9552, -91.6463) knots 0 0 0 1 2 2 2
  spline S81 degree 2 poles (28.9552, -91.6463) (29.3813, -91.6463) (30.0173, -91.8378) (30.3755, -92.0416) knots 0 0 0 1 2 2 2
  line L52 (30.3755, -92.0416) -> (30.4496, -91.7575)
  line L53 (30.4496, -91.7575) -> (32.1662, -91.7575)
  line L54 (32.1662, -91.7575) -> (32.1662, -99.7171)
  line L55 (32.1662, -99.7171) -> (30.3755, -99.7171)
  line L56 (30.3755, -99.7171) -> (30.3755, -96.9013)
  spline S82 degree 2 poles (30.3755, -96.9013) (29.9803, -97.2409) (29.1652, -97.6608) (28.6279, -97.6608) knots 0 0 0 1 2 2 2
  spline S83 degree 2 poles (28.6279, -97.6608) (27.6214, -97.6608) (26.5346, -96.0986) (26.5346, -94.7092) knots 0 0 0 1 2 2 2
  spline S84 degree 2 poles (28.3686, -94.6721) (28.3686, -95.5304) (28.8873, -96.2653) (29.4307, -96.2653) knots 0 0 0 1 2 2 2
  spline S85 degree 2 poles (29.4307, -96.2653) (29.6715, -96.2653) (30.147, -96.1109) (30.3755, -95.9565) knots 0 0 0 1 2 2 2
  line L57 (30.3755, -95.9565) -> (30.3755, -93.079)
  spline S86 degree 2 poles (30.3755, -93.079) (30.1964, -93.0049) (29.8321, -92.9555) (29.653, -92.9555) knots 0 0 0 1 2 2 2
  spline S87 degree 2 poles (29.653, -92.9555) (29.0046, -92.9555) (28.3686, -93.8138) (28.3686, -94.6721) knots 0 0 0 1 2 2 2
  line L58 (20.1867, -97.5065) -> (23.0828, -89.6518)
  line L59 (23.0828, -89.6518) -> (25.0094, -89.6518)
  line L60 (25.0094, -89.6518) -> (24.1387, -91.8995)
  line L61 (24.1387, -91.8995) -> (26.2444, -97.5065)
  line L62 (26.2444, -97.5065) -> (24.3672, -97.5065)
  line L63 (24.3672, -97.5065) -> (23.1569, -93.9002)
  line L64 (23.1569, -93.9002) -> (22.0268, -97.5065)
  line L65 (22.0268, -97.5065) -> (20.1867, -97.5065)
  line L66 (72.9277, -78.9951) -> (75.2557, -78.9951)
  line L67 (75.2557, -78.9951) -> (77.3737, -81.7924)
  line L68 (77.3737, -81.7924) -> (78.0653, -81.7924)
  line L69 (78.0653, -81.7924) -> (78.0653, -78.9951)
  line L70 (78.0653, -78.9951) -> (79.9672, -78.9951)
  line L71 (79.9672, -78.9951) -> (79.9672, -86.6151)
  line L72 (79.9672, -86.6151) -> (76.9044, -86.6151)
  spline S88 degree 2 poles (76.9044, -86.6151) (76.2684, -86.6151) (75.3298, -86.4545) (74.9284, -86.2075) knots 0 0 0 1 2 2 2
  spline S89 degree 2 poles (74.9284, -86.2075) (74.5209, -85.9482) (74.0392, -85.1392) (74.0392, -84.5217) knots 0 0 0 1 2 2 2
  spline S90 degree 2 poles (74.0392, -84.5217) (74.0392, -83.651) (74.8296, -82.5581) (75.4903, -82.237) knots 0 0 0 1 2 2 2
  line L73 (75.4903, -82.237) -> (72.9277, -78.9951)
  spline S91 degree 2 poles (76.0029, -84.2809) (76.0029, -84.5711) (76.2252, -84.9849) (76.4783, -85.096) knots 0 0 0 1 2 2 2
  spline S92 degree 2 poles (76.4783, -85.096) (76.6574, -85.1701) (77.0958, -85.2133) (77.4231, -85.2133) knots 0 0 0 1 2 2 2
  line L74 (77.4231, -85.2133) -> (78.0653, -85.2133)
  line L75 (78.0653, -85.2133) -> (78.0653, -83.1632)
  line L76 (78.0653, -83.1632) -> (77.5157, -83.1632)
  spline S93 degree 2 poles (77.5157, -83.1632) (77.1205, -83.1632) (76.5586, -83.262) (76.3672, -83.4164) knots 0 0 0 1 2 2 2
  spline S94 degree 2 poles (76.3672, -83.4164) (76.1819, -83.5646) (76.0029, -83.9598) (76.0029, -84.2809) knots 0 0 0 1 2 2 2
  spline S95 degree 2 poles (66.9503, -81.8665) (66.9503, -80.4462) (68.5002, -78.816) (69.9143, -78.816) knots 0 0 0 1 2 2 2
  spline S96 degree 2 poles (69.9143, -78.816) (71.3222, -78.816) (72.8845, -80.4462) (72.8845, -81.8665) knots 0 0 0 1 2 2 2
  spline S97 degree 2 poles (72.8845, -81.8665) (72.8845, -83.2991) (71.3222, -84.9231) (69.9143, -84.9231) knots 0 0 0 1 2 2 2
  spline S98 degree 2 poles (69.9143, -84.9231) (68.5064, -84.9231) (66.9503, -83.2929) (66.9503, -81.8665) knots 0 0 0 1 2 2 2
  spline S99 degree 2 poles (68.7842, -81.8541) (68.7842, -82.3666) (68.951, -83.0521) (69.0992, -83.2558) knots 0 0 0 1 2 2 2
  spline S100 degree 2 poles (69.0992, -83.2558) (69.2597, -83.472) (69.6611, -83.6387) (69.9143, -83.6387) knots 0 0 0 1 2 2 2
  spline S101 degree 2 poles (69.9143, -83.6387) (70.1613, -83.6387) (70.5503, -83.4905) (70.7109, -83.2805) knots 0 0 0 1 2 2 2
  spline S102 degree 2 poles (70.7109, -83.2805) (70.8652, -83.0829) (71.0505, -82.3852) (71.0505, -81.8541) knots 0 0 0 1 2 2 2
  spline S103 degree 2 poles (71.0505, -81.8541) (71.0505, -81.3292) (70.8776, -80.6809) (70.7356, -80.4833) knots 0 0 0 1 2 2 2
  spline S104 degree 2 poles (70.7356, -80.4833) (70.5935, -80.2856) (70.1613, -80.1004) (69.9019, -80.1004) knots 0 0 0 1 2 2 2
  spline S105 degree 2 poles (69.9019, -80.1004) (69.6858, -80.1004) (69.2412, -80.2856) (69.1053, -80.4709) knots 0 0 0 1 2 2 2
  spline S106 degree 2 poles (69.1053, -80.4709) (68.951, -80.687) (68.7842, -81.3107) (68.7842, -81.8541) knots 0 0 0 1 2 2 2
  spline S107 degree 2 poles (60.3677, -81.9467) (60.3677, -80.5759) (61.757, -78.8839) (62.7883, -78.8839) knots 0 0 0 1 2 2 2
  spline S108 degree 2 poles (62.7883, -78.8839) (63.2144, -78.8839) (63.8504, -79.0753) (64.2085, -79.2791) knots 0 0 0 1 2 2 2
  line L77 (64.2085, -79.2791) -> (64.2826, -78.9951)
  line L78 (64.2826, -78.9951) -> (65.9993, -78.9951)
  line L79 (65.9993, -78.9951) -> (65.9993, -86.9547)
  line L80 (65.9993, -86.9547) -> (64.2085, -86.9547)
  line L81 (64.2085, -86.9547) -> (64.2085, -84.1389)
  spline S109 degree 2 poles (64.2085, -84.1389) (63.8133, -84.4785) (62.9982, -84.8984) (62.461, -84.8984) knots 0 0 0 1 2 2 2
  spline S110 degree 2 poles (62.461, -84.8984) (61.4545, -84.8984) (60.3677, -83.3361) (60.3677, -81.9467) knots 0 0 0 1 2 2 2
  spline S111 degree 2 poles (62.2016, -81.9097) (62.2016, -82.768) (62.7203, -83.5028) (63.2638, -83.5028) knots 0 0 0 1 2 2 2
  spline S112 degree 2 poles (63.2638, -83.5028) (63.5046, -83.5028) (63.9801, -83.3485) (64.2085, -83.1941) knots 0 0 0 1 2 2 2
  line L82 (64.2085, -83.1941) -> (64.2085, -80.3165)
  spline S113 degree 2 poles (64.2085, -80.3165) (64.0295, -80.2424) (63.6651, -80.193) (63.4861, -80.193) knots 0 0 0 1 2 2 2
  spline S114 degree 2 poles (63.4861, -80.193) (62.8377, -80.193) (62.2016, -81.0514) (62.2016, -81.9097) knots 0 0 0 1 2 2 2
  spline S115 degree 2 poles (53.853, -78.8592) (54.7298, -78.8592) (56.0513, -79.1988) (56.6194, -79.4458) knots 0 0 0 1 2 2 2
  line L83 (56.6194, -79.4458) -> (56.6194, -81.2613)
  line L84 (56.6194, -81.2613) -> (56.4465, -81.2613)
  spline S116 degree 2 poles (56.4465, -81.2613) (55.8722, -80.7735) (54.4952, -80.2486) (53.8468, -80.2486) knots 0 0 0 1 2 2 2
  spline S117 degree 2 poles (53.8468, -80.2486) (53.6801, -80.2486) (53.1429, -80.3227) (52.9823, -80.3968) knots 0 0 0 1 2 2 2
  spline S118 degree 2 poles (52.9823, -80.3968) (52.7847, -80.4833) (52.5068, -80.7982) (52.5068, -81.0514) knots 0 0 0 1 2 2 2
  spline S119 degree 2 poles (52.5068, -81.0514) (52.5068, -81.3416) (52.9576, -81.6997) (53.2664, -81.78) knots 0 0 0 1 2 2 2
  spline S120 degree 2 poles (53.2664, -81.78) (53.6554, -81.885) (54.5384, -82.0641) (54.9274, -82.1999) knots 0 0 0 1 2 2 2
  spline S121 degree 2 poles (54.9274, -82.1999) (55.8105, -82.5087) (56.5762, -83.5646) (56.5762, -84.355) knots 0 0 0 1 2 2 2
  spline S122 degree 2 poles (56.5762, -84.355) (56.5762, -85.4233) (54.7669, -86.7509) (53.4084, -86.7509) knots 0 0 0 1 2 2 2
  spline S123 degree 2 poles (53.4084, -86.7509) (52.7291, -86.7509) (51.383, -86.473) (50.8519, -86.2384) knots 0 0 0 1 2 2 2
  line L85 (50.8519, -86.2384) -> (50.8519, -84.497)
  line L86 (50.8519, -84.497) -> (51.0186, -84.497)
  spline S124 degree 2 poles (51.0186, -84.497) (51.4447, -84.8614) (52.6674, -85.3615) (53.3096, -85.3615) knots 0 0 0 1 2 2 2
  spline S125 degree 2 poles (53.3096, -85.3615) (53.5628, -85.3615) (53.958, -85.2874) (54.1803, -85.1886) knots 0 0 0 1 2 2 2
  spline S126 degree 2 poles (54.1803, -85.1886) (54.3593, -85.1084) (54.6187, -84.7873) (54.6187, -84.5897) knots 0 0 0 1 2 2 2
  spline S127 degree 2 poles (54.6187, -84.5897) (54.6187, -84.2933) (54.205, -83.9536) (53.6122, -83.8178) knots 0 0 0 1 2 2 2
  spline S128 degree 2 poles (53.6122, -83.8178) (53.2293, -83.7313) (52.5192, -83.5646) (52.1116, -83.4226) knots 0 0 0 1 2 2 2
  spline S129 degree 2 poles (52.1116, -83.4226) (51.3212, -83.1323) (50.5493, -82.169) (50.5493, -81.3786) knots 0 0 0 1 2 2 2
  spline S130 degree 2 poles (50.5493, -81.3786) (50.5493, -80.2424) (52.3339, -78.8592) (53.853, -78.8592) knots 0 0 0 1 2 2 2
  spline S131 degree 2 poles (47.4742, -78.8839) (48.5672, -78.8839) (49.5675, -79.7855) (49.5675, -80.8105) knots 0 0 0 1 2 2 2
  line L87 (49.5675, -80.8105) -> (49.5675, -83.4967)
  line L88 (49.5675, -83.4967) -> (50.2529, -83.4967)
  line L89 (50.2529, -83.4967) -> (50.2529, -84.744)
  line L90 (50.2529, -84.744) -> (49.5675, -84.744)
  line L91 (49.5675, -84.744) -> (49.5675, -86.3866)
  line L92 (49.5675, -86.3866) -> (47.7767, -86.3866)
  line L93 (47.7767, -86.3866) -> (47.7767, -84.744)
  line L94 (47.7767, -84.744) -> (46.0477, -84.744)
  line L95 (46.0477, -84.744) -> (46.0477, -83.4967)
  line L96 (46.0477, -83.4967) -> (47.7767, -83.4967)
  line L97 (47.7767, -83.4967) -> (47.7767, -81.4527)
  spline S132 degree 2 poles (47.7767, -81.4527) (47.7767, -81.1502) (47.7644, -80.6994) (47.6903, -80.5203) knots 0 0 0 1 2 2 2
  spline S133 degree 2 poles (47.6903, -80.5203) (47.6162, -80.3412) (47.2519, -80.1313) (46.9061, -80.1313) knots 0 0 0 1 2 2 2
  spline S134 degree 2 poles (46.9061, -80.1313) (46.7579, -80.1313) (46.2947, -80.2548) (46.2021, -80.3042) knots 0 0 0 1 2 2 2
  line L98 (46.2021, -80.3042) -> (46.0477, -80.3042)
  line L99 (46.0477, -80.3042) -> (46.0477, -79.0445)
  spline S135 degree 2 poles (46.0477, -79.0445) (46.338, -78.9704) (46.9925, -78.8839) (47.4742, -78.8839) knots 0 0 0 1 2 2 2
  spline S136 degree 2 poles (42.3736, -78.8407) (44.0038, -78.8407) (45.739, -80.3968) (45.739, -81.8356) knots 0 0 0 1 2 2 2
  spline S137 degree 2 poles (45.739, -81.8356) (45.739, -83.2435) (44.1211, -84.9231) (42.6638, -84.9231) knots 0 0 0 1 2 2 2
  spline S138 degree 2 poles (42.6638, -84.9231) (41.3485, -84.9231) (40.0147, -83.4967) (40.0147, -82.1752) knots 0 0 0 1 2 2 2
  line L100 (40.0147, -82.1752) -> (40.0147, -81.5268)
  line L101 (40.0147, -81.5268) -> (43.9482, -81.5268)
  spline S139 degree 2 poles (43.9482, -81.5268) (43.9235, -81.1255) (43.6333, -80.5944) (43.3986, -80.4339) knots 0 0 0 1 2 2 2
  spline S140 degree 2 poles (43.3986, -80.4339) (43.1702, -80.2733) (42.5527, -80.1374) (42.1883, -80.1374) knots 0 0 0 1 2 2 2
  spline S141 degree 2 poles (42.1883, -80.1374) (41.8796, -80.1374) (41.2744, -80.2733) (41.0213, -80.3906) knots 0 0 0 1 2 2 2
  spline S142 degree 2 poles (41.0213, -80.3906) (40.799, -80.4833) (40.4285, -80.7117) (40.3111, -80.7982) knots 0 0 0 1 2 2 2
  line L102 (40.3111, -80.7982) -> (40.1197, -80.7982)
  line L103 (40.1197, -80.7982) -> (40.1197, -79.3162)
  spline S143 degree 2 poles (40.1197, -79.3162) (40.342, -79.2297) (40.7002, -79.0815) (41.0213, -79.0074) knots 0 0 0 1 2 2 2
  spline S144 degree 2 poles (41.0213, -79.0074) (41.3115, -78.9271) (41.929, -78.8407) (42.3736, -78.8407) knots 0 0 0 1 2 2 2
  spline S145 degree 2 poles (41.7808, -82.6075) (41.7931, -83.1756) (42.2933, -83.7745) (42.8058, -83.7745) knots 0 0 0 1 2 2 2
  spline S146 degree 2 poles (42.8058, -83.7745) (43.3307, -83.7745) (43.9235, -83.1447) (43.9544, -82.6075) knots 0 0 0 1 2 2 2
  line L104 (43.9544, -82.6075) -> (41.7808, -82.6075)
  spline S147 degree 2 poles (36.1491, -78.8407) (37.7794, -78.8407) (39.5145, -80.3968) (39.5145, -81.8356) knots 0 0 0 1 2 2 2
  spline S148 degree 2 poles (39.5145, -81.8356) (39.5145, -83.2435) (37.8967, -84.9231) (36.4394, -84.9231) knots 0 0 0 1 2 2 2
  spline S149 degree 2 poles (36.4394, -84.9231) (35.1241, -84.9231) (33.7903, -83.4967) (33.7903, -82.1752) knots 0 0 0 1 2 2 2
  line L105 (33.7903, -82.1752) -> (33.7903, -81.5268)
  line L106 (33.7903, -81.5268) -> (37.7238, -81.5268)
  spline S150 degree 2 poles (37.7238, -81.5268) (37.6991, -81.1255) (37.4089, -80.5944) (37.1742, -80.4339) knots 0 0 0 1 2 2 2
  spline S151 degree 2 poles (37.1742, -80.4339) (36.9457, -80.2733) (36.3282, -80.1374) (35.9639, -80.1374) knots 0 0 0 1 2 2 2
  spline S152 degree 2 poles (35.9639, -80.1374) (35.6551, -80.1374) (35.05, -80.2733) (34.7968, -80.3906) knots 0 0 0 1 2 2 2
  spline S153 degree 2 poles (34.7968, -80.3906) (34.5745, -80.4833) (34.204, -80.7117) (34.0867, -80.7982) knots 0 0 0 1 2 2 2
  line L107 (34.0867, -80.7982) -> (33.8953, -80.7982)
  line L108 (33.8953, -80.7982) -> (33.8953, -79.3162)
  spline S154 degree 2 poles (33.8953, -79.3162) (34.1176, -79.2297) (34.4757, -79.0815) (34.7968, -79.0074) knots 0 0 0 1 2 2 2
  spline S155 degree 2 poles (34.7968, -79.0074) (35.087, -78.9271) (35.7045, -78.8407) (36.1491, -78.8407) knots 0 0 0 1 2 2 2
  spline S156 degree 2 poles (35.5563, -82.6075) (35.5687, -83.1756) (36.0689, -83.7745) (36.5814, -83.7745) knots 0 0 0 1 2 2 2
  spline S157 degree 2 poles (36.5814, -83.7745) (37.1063, -83.7745) (37.6991, -83.1447) (37.73, -82.6075) knots 0 0 0 1 2 2 2
  line L109 (37.73, -82.6075) -> (35.5563, -82.6075)
  line L110 (31.0794, -78.9951) -> (32.8702, -78.9951)
  line L111 (32.8702, -78.9951) -> (32.8702, -86.9547)
  line L112 (32.8702, -86.9547) -> (31.0794, -86.9547)
  line L113 (31.0794, -86.9547) -> (31.0794, -78.9951)
  spline S158 degree 2 poles (26.7631, -78.8407) (28.3933, -78.8407) (30.1285, -80.3968) (30.1285, -81.8356) knots 0 0 0 1 2 2 2